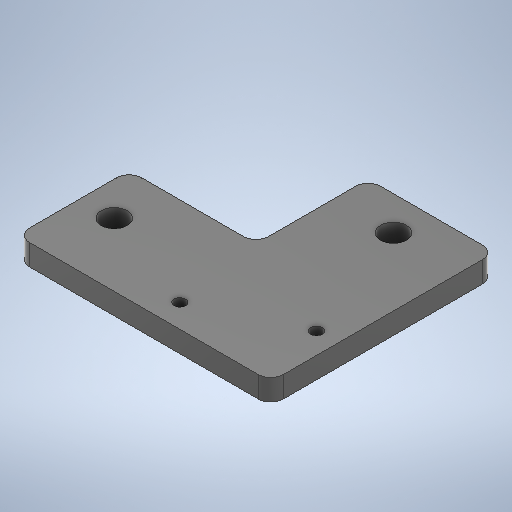
# Autodesk Inventor part: Limit SW Bracket Left
Saved by Autodesk Inventor 2026.2 (Build 302298010, 298A)
## iProperties
Created: 2026-05-06
Part Number: Limit SW Bracket Left
Material: ABS Plastic
Document SubType Name: Modeling
Designer: chanh
Density: 1.06 g/cm^3
Appearance: Smooth - White
Author: chanh
Autodesk Inventor part; units mm, degrees
ref_plane "YZ Plane" through (0, 0, 0) normal (1, 0, 0) x (0, 1, 0)
ref_plane "XZ Plane" through (0, 0, 0) normal (0, 1, 0) x (-1, 0, 0)
ref_plane "XY Plane" through (0, 0, 0) normal (0, 0, 1) x (1, 0, 0)
sketch "Sketch1" plane through (0, 0, 0) normal (0, 1, 0) x (-1, 0, 0)
  line L0 (30, -26.5) -> (-30, -26.5)
  line L1 (-30, -26.5) -> (-30, 26.5)
  line L2 (-30, 26.5) -> (30, 26.5)
  line L3 (30, 26.5) -> (30, -26.5)
  line L4 (30, -26.5) -> (-30, 26.5) construction
  line L5 (-30, -26.5) -> (30, 26.5) construction
  line L6 (-3, 21) -> (-25, 21) construction
  line L7 (-25, 21) -> (-25, 10.7) construction
  line L8 (-25, 10.7) -> (-3, 10.7) construction
  line L9 (-3, 10.7) -> (-3, 21) construction
  line L10 (0, 0) -> (30, 0)
  line L11 (0, 0) -> (0, -26.5)
  point P0 (-14, -18.5)
  point P1 (-14, 10.7)
  point P2 (22, 11.5)
  dimension "d0" = 60
  dimension "d1" = 53
  dimension "d2" = 5
  dimension "d3" = 5.5
  dimension "d4" = 22
  dimension "d5" = 10.3
  dimension "d6" = 45
  dimension "d7" = 8
  dimension "d8" = 15
  constraints: 24 end point, 5 midpoint, 4 parallel, 2 coincident, 2 horizontal, 2 perpendicular, 1 vertical alignment
  measures "d0" distance of L1.end L2.end
  measures "d1" distance of L0.end L1.end
  measures "d2" distance between parallel lines of L1 L7
  measures "d3" distance between parallel lines of L2 L6
  measures "d4" distance between parallel lines of L7 L9
  measures "d5" distance between parallel lines of L8 L6
  measures "d6" distance from line of point (-14, -18.5) L2
  measures "d7" distance from line of L3 point (22, 11.5)
  measures "d8" distance from line of L2 point (22, 11.5)
extrude "Extrusion1" add sketch "Sketch1" along normal blind 5 contours L0 L1 L2 L3 L10 L11
hole "Hole1" at (3, 0, 21) at (25, 0, 10.7) direction (0, 1, 0) diameter 2.7 end through all
hole "Hole2" at (14, 0, -18.5) at (-22, 0, 11.5) direction (0, 1, 0) diameter 6.1 end through all
fillet "Fillet1" radius 3 6 edges at (-30, 2.5, 26.5) (30, 2.5, 26.5) (30, 2.5, -26.5) (0, 2.5, -26.5) (0, 2.5, 0) (-30, 2.5, 0)
body "Solid1"
